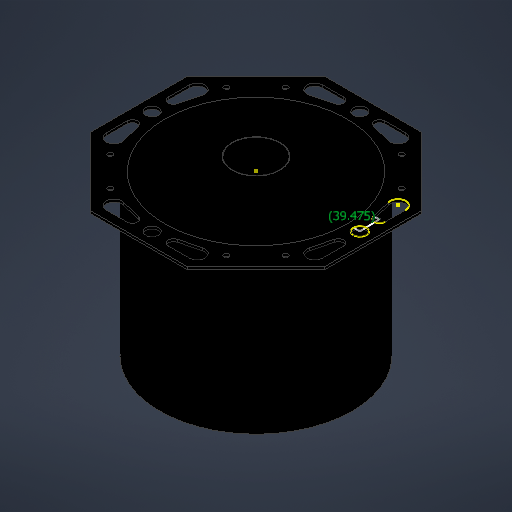
# Autodesk Inventor part: Telescope_Base
Saved by Autodesk Inventor 2026.2 (Build 302298000, 298)
## iProperties
Created: 2025-12-10
Part Number: Telescope_Base
Material: Generic
Document SubType Name: Modeling
Designer: Thoma
Density: 1 g/cm^3
Appearance: Default
Author: Thoma
Autodesk Inventor part; units mm, degrees
ref_plane "YZ Plane" through (0, 0, 0) normal (1, 0, 0) x (0, 1, 0)
ref_plane "XZ Plane" through (0, 0, 0) normal (0, 1, 0) x (-1, 0, 0)
ref_plane "XY Plane" through (0, 0, 0) normal (0, 0, 1) x (1, 0, 0)
sketch "Sketch1" plane through (0, 0, 0) normal (0, 1, 0) x (-1, 0, 0)
  line L0 (-92.5, -223.3148) -> (-223.3148, -92.5)
  line L1 (-223.3148, -92.5) -> (-223.3148, 92.5)
  line L2 (-223.3148, 92.5) -> (-92.5, 223.3148)
  line L3 (-92.5, 223.3148) -> (92.5, 223.3148)
  line L4 (92.5, 223.3148) -> (223.3148, 92.5)
  line L5 (223.3148, 92.5) -> (223.3148, -92.5)
  line L6 (223.3148, -92.5) -> (92.5, -223.3148)
  line L7 (92.5, -223.3148) -> (-92.5, -223.3148)
  circle A0 centre (0, 0) radius 46
  circle A1 centre (0, 0) radius 174
  dimension "d0" = 185
  dimension "d1" = 128
  dimension "d2" = 92
  constraints: 16 end point, 3 coincident, 2 centre point, 17 other
  measures "d0" distance of L5.end L4.end
  measures "d1" radial gap between concentric circles of A1 A0
  measures "d2" diameter of A0
extrude "Extrusion1" add sketch "Sketch1" along normal blind 5
sketch "Sketch2" plane through (0, 5, 0) normal (0, 1, 0) x (1, 0, 0)
  circle A0 centre (0, 0) radius 46
  constraints: 1 centre point, 1 coincident
extrude "Extrusion2" add sketch "Sketch2" against normal blind 300
sketch "Sketch3" plane through (0, -295, 0) normal (0, -1, 0) x (-1, 0, 0)
  circle A0 centre (0, 0) radius 45
  dimension "d9" = 90
  constraints: 1 centre point, 1 coincident
  measures "d9" diameter of A0
extrude "Extrusion3" cut sketch "Sketch3" against normal blind 300
sketch "Sketch4" plane through (0, 5, 0) normal (0, 1, 0) x (1, 0, 0)
  circle A0 centre (0, 0) radius 174 projected
  line L0 (0, 174) -> (0, 223.3148)
  line L1 (92.5, 223.3148) -> (-92.5, 223.3148) projected
  circle A1 centre (0, 198.6574) radius 12.5
  dimension "d10" = 25
  constraints: 2 end point, 2 midpoint, 1 centre point, 1 vertical, 1 vertical alignment, 1 other
  measures "d10" diameter of A1
extrude "Extrusion4" cut sketch "Sketch4" against normal blind 5 contours A1 L0 | L0 A1
pattern_circular "Circular Pattern1" count 4 over 360 about axis through (0, -10, 0) along (0, 1, 0) of "Extrusion4"
sketch "Sketch5" plane through (0, 5, 0) normal (0, 1, 0) x (1, 0, 0)
  line L0 (-223.3148, -92.5) -> (-92.5, -223.3148) projected
  line L1 (-92.5, -223.3148) -> (-66.5869, -160.755)
  circle A0 centre (0, 0) radius 174 projected
  circle A1 centre (-79.5435, -192.0349) radius 15
  line L2 (-92.5, -223.3148) -> (92.5, -223.3148) projected
  circle A2 centre (0, -198.6574) radius 12.5 projected
  line L3 (0, -211.1574) -> (0, -186.1574)
  line L4 (-44.7395, -223.3148) -> (-34.1805, -170.6098)
  line L5 (92.5, -223.3148) -> (223.3148, -92.5) projected
  line L6 (92.5, -223.3148) -> (66.5869, -160.755)
  circle A3 centre (79.5435, -192.0349) radius 15
  arc A4 (-79.5435, -192.0349) -> (79.5435, -192.0349) centre (0, 282.3572) ccw
  circle A5 centre (-39.4746, -197.0349) radius 10
  circle A6 centre (39.4746, -197.0349) radius 10
  line L7 (-79.5435, -207.0349) -> (-39.4746, -207.0349)
  line L8 (-79.5435, -192.0349) -> (-39.4746, -197.0349)
  line L9 (-75.8573, -177.4949) -> (-37.0171, -187.3415)
  dimension "d16" = 30
  dimension "d18" = 20
  dimension "d17" = 30
  constraints: 14 end point, 9 point on circle, 3 centre point, 3 horizontal, 3 line through centre, 3 symmetric about line, 2 midpoint, 2 point on line, 1 vertical, 7 other
  measures "d17" diameter of A3
extrude "Extrusion5" cut sketch "Sketch5" against normal blind 5 contours A1 L1 | L1 A4 A1 | L8 A1 A4 | L1 A1 L8 | L9 L1 A1 | A1 A4 A5 L4 L7 | L4 A5 L7 | L1 L9 L4 A5 L8 A1 | A1 L8 A5 A4 | A5 A4 L4 | L4 A4 A5 | A5 L8 A4 | A5 L4 L8 | L9 A5 L4 | L4 A5 A4
mirror "Mirror1" about plane through (0, 0, 0) normal (1, 0, 0) of "Extrusion5"
pattern_circular "Circular Pattern2" count 4 over 360 about axis through (0, -10, 0) along (0, 1, 0) of "Extrusion5", "Mirror1"
sketch "Sketch6" plane through (0, 5, 0) normal (0, 1, 0) x (1, 0, 0)
  arc A0 (177.4949, -75.8573) -> (207.0349, -79.5435) centre (192.0349, -79.5435) ccw projected
  line L0 (207.0349, -79.5435) -> (207.0349, -39.4746) projected
  line L1 (207.0349, -79.5435) -> (177.0349, -79.5435)
  arc A1 (79.5435, -207.0349) -> (75.8573, -177.4949) centre (79.5435, -192.0349) ccw projected
  line L2 (75.8573, -177.4949) -> (79.5435, -192.0349)
  line L3 (0, 0) -> (79.5435, -79.5435)
  line L4 (92.5, -223.3148) -> (223.3148, -92.5) projected
  line L5 (92.5, -223.3148) -> (223.3148, -92.5) projected
  line L6 (79.5435, -79.5435) -> (157.9074, -157.9074)
  circle A2 centre (0, 0) radius 174 projected
  line L7 (123.0366, -123.0366) -> (157.9074, -157.9074)
  arc A3 (79.5435, -192.0349) -> (140.472, -140.472) centre (-199.6567, 199.6567) ccw
  arc A4 (140.472, -140.472) -> (192.0349, -79.5435) centre (-199.6567, 199.6567) ccw
  circle A5 centre (167.5194, -111.0791) radius 5
  dimension "d26" = 10
  dimension "d27" = 481.0145
  constraints: 10 end point, 6 point on circle, 3 centre point, 3 perpendicular, 2 midpoint, 2 point on line, 1 horizontal, 2 other
  measures "d26" diameter of A5
  measures "d27" radius of A3
extrude "Extrusion6" cut sketch "Sketch6" against normal blind 5 contours A5 A4 | A4 A5
mirror "Mirror2" about plane through (0, 0, 0) normal (0, 0, 1) of "Extrusion6"
pattern_circular "Circular Pattern3" count 4 over 360 about axis through (0, -10, 0) along (0, 1, 0) of "Extrusion6", "Mirror2"
sketch "Sketch7" plane through (0, 5, 0) normal (0, 1, 0) x (1, 0, 0)
  arc A0 (207.0349, 79.5435) -> (177.4949, 75.8573) centre (192.0349, 79.5435) ccw projected
  circle A1 centre (198.6574, 0) radius 12.5 projected
  line L0 (186.1574, 0) -> (198.6574, 0)
  arc A2 (187.3415, 37.0171) -> (207.0349, 39.4746) centre (197.0349, 39.4746) ccw projected
  line L1 (187.3415, 37.0171) -> (197.0349, 39.4746)
  line L2 (198.6574, 0) -> (197.0349, 39.4746)
  point P0 (0, 0)
  dimension "d33" = 39.4746
  constraints: 6 end point, 1 horizontal, 1 horizontal alignment, 1 other
  measures "d33" vertical distance of L0.end L1.end
sketch "Sketch8" plane through (0, 0, 0) normal (0, -1, 0) x (1, 0, 0)
  circle A0 centre (0, 0) radius 184
  circle A1 centre (0, 0) radius 174 projected
  dimension "d34" = 10
  constraints: 1 centre point, 1 coincident
  measures "d34" radial gap between concentric circles of A1 A0
extrude "Extrusion7" add sketch "Sketch8" along normal blind 300
sketch "Sketch9" plane through (0, -300, 0) normal (0, -1, 0) x (1, 0, 0)
  circle A0 centre (0, 0) radius 174
  constraints: 1 centre point, 1 coincident
extrude "Extrusion8" add sketch "Sketch9" against normal blind 2
sketch "Sketch10" plane through (0, 5, 0) normal (0, 1, 0) x (1, 0, 0)
  circle A0 centre (0, 0) radius 45
  circle A1 centre (0, 0) radius 46
  constraints: 2 centre point, 2 coincident
extrude "Extrusion9" add sketch "Sketch10" along normal blind 25
body "Solid1"
